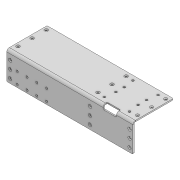
# Autodesk Inventor part: CCM_Mount_E
Saved by Autodesk Inventor 2020 (Build 240168000, 168)
## iProperties
Created: 2021-12-05
Part Number: CCM_Mount_E
Material: 一般
Document SubType Name: Sheet Metal
Designer: ken113
Density: 1 g/cm^3
Sheet Metal Rule: Default_mm
Appearance: 既定
Author: ken113
Autodesk Inventor part; units mm, degrees
ref_plane "YZ Plane" through (0, 0, 0) normal (1, 0, 0) x (0, 1, 0)
ref_plane "XZ Plane" through (0, 0, 0) normal (0, 1, 0) x (-1, 0, 0)
ref_plane "XY Plane" through (0, 0, 0) normal (0, 0, 1) x (1, 0, 0)
sketch "スケッチ1" plane through (0, 0, 0) normal (0, 0, 1) x (1, 0, 0)
  line L0 (150, -33.5) -> (-150, -33.5)
  line L1 (-150, -33.5) -> (-150, 33.5)
  line L2 (-150, 33.5) -> (150, 33.5)
  line L3 (150, 33.5) -> (150, -33.5)
  line L4 (150, -33.5) -> (-150, 33.5) construction
  line L5 (-150, -33.5) -> (150, 33.5) construction
  point P0 (0, 0)
  dimension "d1" = 67
  dimension "d2" = 300
  measures "d1" distance of L2.end L0.start
  measures "d2" distance of L0.start L0.end
extrude "プレート1" add sketch "スケッチ1" along normal blind 3
sketch "スケッチ2" plane through (150, 30.5, 3) normal (0, 1, 0) x (-1, 0, 0)
  line L0 (300, 0) -> (0, 0)
  line L1 (0, 0) -> (0, -96)
  line L2 (0, -96) -> (300, -96)
  line L3 (300, -96) -> (300, 0)
  constraints: 6 end point, 1 horizontal, 1 perpendicular, 1 vertical
edge flange "フランジ1" height 96 angle 90 thickness 3 bend radius 3 thickness toward (0, 1, 0) relief straight relief width 3 relief depth 1.5 edges at (0, 33.5, 0) wall of the first edge with corners at (-150, 30.5, 3) (150, 30.5, 3) (150, 30.5, -93) (-150, 30.5, -93)
bend "曲げ1"
corner "コーナー1"
fillet "フィレット1" radius 2 4 edges at (-150, 32, -93) (150, 32, -93) (150, -33.5, 1.5) (-150, -33.5, 1.5)
sketch "スケッチ3" plane through (-150, 30.5, -3) normal (0, -1, 0) x (1, 0, 0)
  line L0 (81.5, -55) -> (28.5, -55)
  line L1 (28.5, -55) -> (28.5, -35)
  line L2 (28.5, -35) -> (81.5, -35)
  line L3 (81.5, -35) -> (81.5, -55)
  line L4 (81.5, -55) -> (28.5, -35) construction
  line L5 (28.5, -55) -> (81.5, -35) construction
  line L6 (25, -79) -> (85, -79)
  line L7 (85, -79) -> (85, -11)
  line L8 (85, -11) -> (25, -11)
  line L9 (25, -11) -> (25, -79)
  line L10 (25, -79) -> (85, -11) construction
  line L11 (85, -79) -> (25, -11) construction
  line L12 (0, 0) -> (0, -88) projected
  line L13 (2, -90) -> (298, -90) projected
  point P0 (150, 3)
  point P1 (55, -45)
  dimension "d15" = 53
  dimension "d16" = 20
  dimension "d17" = 60
  dimension "d18" = 68
  dimension "d20" = 45
  dimension "d28" = 55
  constraints: 24 end point, 4 midpoint, 4 parallel, 2 horizontal, 2 perpendicular
  measures "d15" distance of L1.end L2.end
  measures "d16" distance of L0.end L1.end
  measures "d17" distance of L7.end L8.end
  measures "d18" distance of L6.end L7.end
  measures "d20" distance from line of L13 point (55, -45)
  measures "d28" distance from line of point (55, -45) L12
hole "穴1" at (-125, 30.5, -82) at (-65, 30.5, -82) at (-125, 30.5, -14) at (-65, 30.5, -14) at (-68.5, 30.5, -38) at (-68.5, 30.5, -58) at (-121.5, 30.5, -58) at (-121.5, 30.5, -38) direction (0, 1, 0) diameter 5.2 end through all
sketch "スケッチ4" plane through (-150, 33.5, -3) normal (0, 1, 0) x (1, 0, 0)
  circle A0 centre (28.5, 55) radius 2.6 projected
  circle A1 centre (81.5, 35) radius 2.6 projected
  circle A2 centre (25, 11) radius 2.6 projected
  circle A3 centre (25, 79) radius 2.6 projected
  circle A4 centre (85, 79) radius 2.6 projected
  circle A5 centre (85, 11) radius 2.6 projected
  circle A6 centre (81.5, 55) radius 2.6 projected
  circle A7 centre (28.5, 35) radius 2.6 projected
  arc A8 (300, 88) -> (298, 90) centre (298, 88) ccw projected
  line L0 (2, 90) -> (298, 90) projected
  arc A9 (2, 90) -> (0, 88) centre (2, 88) ccw projected
  line L1 (0, 0) -> (0, 88) projected
  line L2 (0, 0) -> (300, 0) projected
  line L3 (300, 88) -> (300, 0) projected
  line L4 (102, 13) -> (8, 13)
  line L5 (8, 13) -> (8, 80)
  line L6 (8, 80) -> (102, 80)
  line L7 (102, 80) -> (102, 13)
  line L8 (102, 80) -> (292, 80)
  line L9 (292, 80) -> (292, 13)
  line L10 (292, 13) -> (102, 13)
  line L11 (102, 13) -> (102, 80)
  point P0 (150, -3)
  point P1 (292, 46.5)
  point P2 (102, 46.5)
  point P3 (8, 46.5)
  dimension "d29" = 8
  dimension "d30" = 10
  dimension "d31" = 13
  dimension "d39" = 8
  dimension "d40" = 17
  constraints: 16 end point, 4 parallel, 3 midpoint, 2 horizontal, 2 perpendicular, 1 horizontal alignment
  measures "d29" distance between parallel lines of L9 L3
  measures "d30" distance between parallel lines of L6 L0
  measures "d31" distance between parallel lines of L2 L4
  measures "d39" distance between parallel lines of L1 L5
  measures "d40" distance from line of L7 A5.centre
hole "穴2" at (142, 33.5, -49.5) at (-48, 33.5, -49.5) at (-142, 33.5, -49.5) at (142, 33.5, -83) at (-48, 33.5, -83) at (-142, 33.5, -83) at (-142, 33.5, -16) at (-48, 33.5, -16) at (142, 33.5, -16) direction (0, -1, 0) diameter 4.3 end through all countersink diameter 8 countersink angle 90
sketch "スケッチ5" plane through (0, 0, 3) normal (0, 0, 1) x (1, 0, 0)
  arc A0 (-150, -31.5) -> (-148, -33.5) centre (-148, -31.5) ccw projected
  line L0 (148, -33.5) -> (-148, -33.5) projected
  arc A1 (148, -33.5) -> (150, -31.5) centre (148, -31.5) ccw projected
  line L1 (150, 27.5) -> (150, -31.5) projected
  line L2 (150, 27.5) -> (-150, 27.5) projected
  line L3 (-150, -31.5) -> (-150, 27.5) projected
  line L4 (142, 14.5) -> (-142, 14.5)
  line L5 (-142, 14.5) -> (-142, -23.5)
  line L6 (-142, -23.5) -> (142, -23.5)
  line L7 (142, -23.5) -> (142, 14.5)
  line L8 (-142, -23.5) -> (-48, -23.5)
  line L9 (-48, -23.5) -> (-48, 14.5)
  line L10 (-48, 14.5) -> (-142, 14.5)
  line L11 (-142, 14.5) -> (-142, -23.5)
  line L12 (-146, 33.5) -> (-138, 33.5) projected
  line L13 (-52, 33.5) -> (-44, 33.5) projected
  line L14 (138, 33.5) -> (146, 33.5) projected
  point P0 (0, 0)
  point P1 (-48, -4.5)
  point P2 (-142, -4.5)
  point P3 (142, -4.5)
  dimension "d41" = 8
  dimension "d42" = 8
  dimension "d43" = 94
  dimension "d44" = 13
  dimension "d45" = 10
  constraints: 16 end point, 4 parallel, 3 midpoint, 2 horizontal, 2 perpendicular, 1 point on line
  measures "d41" distance between parallel lines of L7 L1
  measures "d42" distance between parallel lines of L3 L5
  measures "d43" distance between parallel lines of L5 L9
  measures "d44" distance between parallel lines of L10 L2
  measures "d45" distance between parallel lines of L0 L6
hole "穴3" at (-48, -4.5, 3) at (-142, -4.5, 3) at (142, -4.5, 3) at (142, 14.5, 3) at (-48, 14.5, 3) at (-142, 14.5, 3) at (-142, -23.5, 3) at (-48, -23.5, 3) at (142, -23.5, 3) direction (0, 0, -1) diameter 4.3 end through all countersink diameter 8 countersink angle 90
sketch "スケッチ6" plane through (0, 0, 0) normal (0, 0, -1) x (-1, 0, 0)
  line L0 (-55, -27) -> (-125, -27)
  line L1 (-125, -27) -> (-125, 0)
  line L2 (-125, 0) -> (-55, 0)
  line L3 (-55, 0) -> (-55, -27)
  line L4 (-55, -27) -> (-125, 0) construction
  line L5 (-125, -27) -> (-55, 0) construction
  line L6 (-148, -33.5) -> (148, -33.5) projected
  line L7 (-150, 27.5) -> (-150, -31.5) projected
  line L8 (-101.6667, -27) -> (-78.3333, -27)
  line L9 (-78.3333, -27) -> (-78.3333, 0)
  line L10 (-78.3333, 0) -> (-101.6667, 0)
  line L11 (-101.6667, 0) -> (-101.6667, -27)
  line L12 (-101.6667, -27) -> (-78.3333, 0) construction
  line L13 (-78.3333, -27) -> (-101.6667, 0) construction
  point P0 (0, 0)
  point P1 (-90, -13.5)
  point P2 (-42.5, -33.5)
  dimension "d53" = 6.5
  dimension "d54" = 27
  dimension "d55" = 25
  dimension "d56" = 107.5
  dimension "d58" = 70
  dimension "d59" = 23.3333
  constraints: 24 end point, 4 midpoint, 4 parallel, 2 coincident, 2 horizontal, 2 perpendicular, 2 point on line
  measures "d53" distance between parallel lines of L6 L0
  measures "d54" distance of L0.end L1.end
  measures "d55" distance between parallel lines of L7 L1
  measures "d56" distance from line of point (-42.5, -33.5) L7
  measures "d58" distance of L0.start L0.end
  measures "d59" distance between parallel lines of L11 L1
hole "穴4" at (55, -27, 0) at (55, 0, 0) at (78.3333, -27, 0) at (78.3333, 0, 0) at (101.6667, 0, 0) at (101.6667, -27, 0) at (125, -27, 0) at (125, 0, 0) direction (0, 0, 1) diameter 5.2 end through all
mirror "ミラー1" about plane through (-150, 30.5, -3) normal (-1, 0, 0) remove original yes
sketch "スケッチ7" plane through (-448, -33.5, 3) normal (0, 0, 1) x (1, 0, 0)
  line L0 (227, 71.7912) -> (259, 71.7912)
  line L1 (259, 71.7912) -> (259, 57)
  line L2 (259, 57) -> (227, 57)
  line L3 (227, 57) -> (227, 71.7912)
  circle A0 centre (196, 48) radius 4 projected
  circle A1 centre (290, 48) radius 4 projected
  circle A2 centre (290, 48) radius 2.15 projected
  line L4 (196, 48) -> (290, 48)
  line L5 (298, 67) -> (-2, 67) projected
  point P0 (448, 33.5)
  point P1 (243, 48)
  point P2 (243, 57)
  point P3 (259, 67)
  point P4 (227, 67)
  dimension "d67" = 32
  dimension "d68" = 10
  constraints: 10 end point, 2 horizontal, 2 midpoint, 2 parallel, 1 perpendicular, 1 vertical alignment
  measures "d67" distance of L0.start L0.end
  measures "d68" distance between parallel lines of L2 L5
extrude "押し出し1" cut sketch "スケッチ7" against normal blind 10 contours L5 L1 L2 L3
fillet "フィレット2" radius 2 4 edges at (-221, 32, -7) (-221, 23.5, 1.5) (-189, 32, -7) (-189, 23.5, 1.5)
equation "\"d26\" = Thickness"
equation "\"d37\" = Thickness"
equation "\"d51\" = Thickness"
equation "\"d59\" = 0.333333 * d58"
equation "\"d65\" = Thickness"
equation "\"d3\" = Thickness"
equation "\"d4\" = BendReliefWidth"
equation "\"d5\" = BendReliefDepth"
equation "\"d6\" = MinimumRemnant"
equation "\"d7\" = TransitionRadius"
equation "\"d10\" = BendRadius"
equation "\"d11\" = CornerReliefSize"
equation "\"d12\" = GapSize"
equation "\"d13\" = JacobiRadiusSize"
equation "\"BendRadius\" = Thickness"
equation "\"BendReliefWidth\" = Thickness"
equation "\"BendReliefDepth\" = 0.5 * Thickness"
equation "\"CornerReliefSize\" = 4 * Thickness"
equation "\"MinimumRemnant\" = 2 * Thickness"
equation "\"TransitionRadius\" = BendRadius"
equation "\"JacobiRadiusSize\" = BendRadius"
equation "\"GapSize\" = Thickness"
equation "\"Thickness\" = 3"
